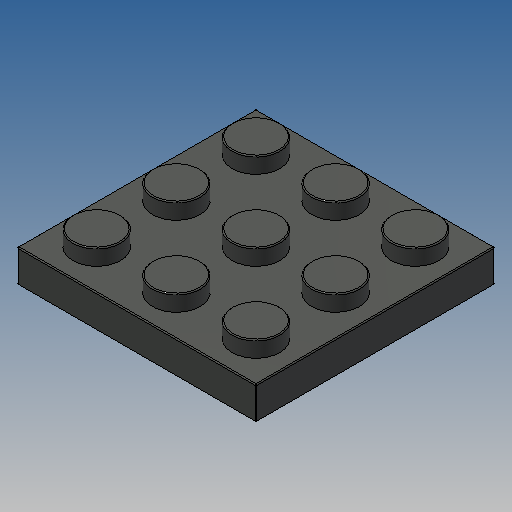
# Autodesk Inventor part: 11212-DkBluishGray
Saved by Autodesk Inventor 2025 (Build 290162010, 162A)
## iProperties
Created: 2014-06-03
Part Number: 11212-DkBluishGray
Material: ABS Plastic
Document SubType Name: Modeling
Designer: D. Kohfeld
Density: 1.06 g/cm^3
Appearance: DkBluishGray
Mass: 1.599 g
Surface Area: 20.2639 cm^2
Volume: 1.50849 cm^3
Author: D. Kohfeld
Autodesk Inventor part; units mm, degrees
ref_plane "YZ Plane" through (0, 0, 0) normal (1, 0, 0) x (0, 1, 0)
ref_plane "XZ Plane" through (0, 0, 0) normal (0, 1, 0) x (-1, 0, 0)
ref_plane "XY Plane" through (0, 0, 0) normal (0, 0, 1) x (1, 0, 0)
sketch "Sketch2" plane through (0, 0, 0) normal (0, 1, 0) x (-1, 0, 0)
  line L0 (-12, 12) -> (12, 12)
  line L1 (12, 12) -> (12, -12)
  line L2 (12, -12) -> (-12, -12)
  line L3 (-12, -12) -> (-12, 12)
  point P0 (0, 0)
  point P1 (0, 12)
  point P2 (-12, 0)
  dimension "d0" = 24
  dimension "d1" = 24
  constraints: 8 end point, 2 midpoint, 2 parallel, 1 horizontal, 1 horizontal alignment, 1 perpendicular, 1 vertical alignment
  measures "d0" distance of L1.end L2.end
  measures "d1" distance of L2.end L0.start
extrude "Extrusion1" add sketch "Sketch2" along normal blind 3.2
sketch "Sketch9" plane through (0, 3.2, 0) normal (0, 1, 0) x (1, 0, 0)
  line L0 (-12, -12) -> (12, -12) projected
  line L1 (-12, 12) -> (-12, -12) projected
  circle A0 centre (-8, -8) radius 2.4
  point P0 (0, 0)
  dimension "d63" = 4.8
  dimension "d64" = 4
  dimension "d65" = 4
  constraints: 1 centre point
  measures "d63" diameter of A0
  measures "d64" distance from line of A0.centre L0
  measures "d65" distance from line of A0.centre L1
extrude "Extrusion4" add sketch "Sketch9" along normal blind 1.6
fillet "Fillet2" radius 0.1 1 edges at (-10.4, 4.8, 8)
pattern_linear "Rectangular Pattern1" count 3 spacing 8 along (1, 0, 0) count 3 spacing 8 along (0, 0, -1) of "Extrusion4", "Fillet2"
sketch "Sketch3" plane through (0, 0, 0) normal (0, -1, 0) x (1, 0, 0)
  line L0 (12, 12) -> (-12, 12) projected
  line L1 (-12, 12) -> (-12, -12) projected
  line L2 (-10.4, 10.4) -> (10.4, 10.4)
  line L3 (10.4, 10.4) -> (10.4, -10.4)
  line L4 (10.4, -10.4) -> (-10.4, -10.4)
  line L5 (-10.4, -10.4) -> (-10.4, 10.4)
  circle A0 centre (-4, -4) radius 3.2569
  circle A1 centre (-4, -4) radius 2.4
  line L6 (-12, -12) -> (12, -12) projected
  point P0 (0, 0)
  point P1 (-10.4, 0)
  point P2 (0, 10.4)
  dimension "d8" = 1.6
  dimension "d60" = 6.5137
  dimension "d61" = 4.8
  dimension "d62" = 1.6
  dimension "d75" = 8
  dimension "d76" = 8
  constraints: 8 end point, 2 centre point, 2 midpoint, 2 parallel, 1 coincident, 1 horizontal, 1 horizontal alignment, 1 perpendicular, 1 vertical alignment
  measures "d8" distance between parallel lines of L1 L5
  measures "d60" diameter of A0
  measures "d61" diameter of A1
  measures "d62" distance between parallel lines of L0 L2
  measures "d75" distance from line of A0.centre L1
  measures "d76" distance from line of A0.centre L6
extrude "Extrusion2" cut sketch "Sketch3" against normal blind 1.6 contours L2 L3 L4 L5 | A0 | A1
extrude "Extrusion5" add sketch "Sketch3" against normal up to next contours A0
pattern_linear "Rectangular Pattern2" count 2 spacing 8 along (1, 0, 0) count 2 spacing 8 along (0, 0, 1) of "Extrusion5"
fillet "Fillet1" radius 0.1 8 edges at (-12, 1.6, 12) (0, 3.2, 12) (-12, 3.2, 0) (12, 1.6, 12) (12, 3.2, 0) (0, 3.2, -12) (12, 1.6, -12) (-12, 1.6, -12)
equation "\"d4\" = 0.333333 * lh"
equation "\"d63\" = kd"
equation "\"d64\" = 0.5 * lu"
equation "\"d65\" = d64"
equation "\"d66\" = knobh"
equation "\"d71\" = lu"
equation "\"d74\" = lu"
equation "\"d8\" = d62"
equation "\"d60\" = tubeod"
equation "\"d61\" = kd"
equation "\"d62\" = wall"
equation "\"d75\" = lu"
equation "\"d76\" = d75"
equation "\"d11\" = 0.333333 * lh - topthk"
equation "\"d81\" = lu"
equation "\"d84\" = lu"
equation "\"lh\" = 9.6"
equation "\"kd\" = 4.8"
equation "\"lu\" = 8"
equation "\"knobh\" = 1.6"
equation "\"tubeod\" = 6.513708"
equation "\"wall\" = 1.6"
equation "\"topthk\" = 1.6"
body "Solid1"
